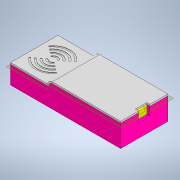
# Autodesk Inventor part: Part1
Saved by Autodesk Inventor 2021 (Build 250183000, 183)
## iProperties
Created: 2026-03-20
Part Number: Part1
Material: Generic
Document SubType Name: Modeling
Designer: Ignacio
Density: 1 g/cm^3
Appearance: Default
Author: Ignacio
Autodesk Inventor part; units mm, degrees
ref_plane "YZ Plane" through (0, 0, 0) normal (1, 0, 0) x (0, 1, 0)
ref_plane "XZ Plane" through (0, 0, 0) normal (0, 1, 0) x (-1, 0, 0)
ref_plane "XY Plane" through (0, 0, 0) normal (0, 0, 1) x (1, 0, 0)
sketch "Sketch1" plane through (0, 0, 0) normal (0, 1, 0) x (-1, 0, 0)
  line L0 (0, 0) -> (51, 0)
  line L1 (51, 0) -> (51, -51)
  line L2 (51, -51) -> (0, -51)
  line L3 (0, -51) -> (0, 0)
  dimension "d0" = 51
  constraints: 8 end point, 2 parallel, 2 perpendicular, 1 horizontal
  measures "d0" distance of L0.end L1.end
extrude "Extrusion1" add sketch "Sketch1" along normal blind 1.6
sketch "Sketch2" plane through (0, 0, 0) normal (0, -1, 0) x (1, 0, 0)
  line L0 (-49, -2) -> (-2, -2)
  line L1 (-2, -2) -> (-2, -49)
  line L2 (-2, -49) -> (-49, -49)
  line L3 (-49, -49) -> (-49, -2)
  line L4 (-49, -2) -> (-2, -49) construction
  line L5 (-2, -2) -> (-49, -49) construction
  line L6 (0, 0) -> (0, -51) construction
  line L7 (0, -25.5) -> (-25.5, -25.5) construction
  line L8 (-25.5, -25.5) -> (-25.5, -51) construction
  line L9 (0, -51) -> (-51, -51) construction
  dimension "d3" = 2
  dimension "d4" = 2
  constraints: 16 end point, 4 midpoint, 3 perpendicular, 2 parallel, 1 horizontal
  measures "d3" distance between parallel lines of L6 L1
  measures "d4" distance between parallel lines of L9 L2
extrude "Extrusion2" add sketch "Sketch2" along normal blind 4
sketch "Sketch3" plane through (0, 0, 0) normal (1, 0, 0) x (0, 1, 0)
  line L0 (1.6, -51) -> (1.6, 0) projected
  line L1 (1.6, -9.85) -> (16.1, -9.85)
  line L2 (16.1, -9.85) -> (16.1, -41.15)
  line L3 (16.1, -41.15) -> (1.6, -41.15)
  line L4 (1.6, -41.15) -> (1.6, -9.85)
  line L5 (1.6, -25.5) -> (16.1, -25.5) construction
  point P0 (0, 0)
  point P1 (1.6, -41.15)
  dimension "d7" = 14.5
  dimension "d8" = 31.3
  constraints: 10 end point, 3 midpoint, 2 parallel, 1 horizontal, 1 perpendicular, 1 point on line
  measures "d7" distance of L2.end L3.end
  measures "d8" distance of L1.end L2.end
extrude "Extrusion3" add sketch "Sketch3" along normal blind 15.4 and the other way blind 42
sketch "Sketch4" plane through (15.4, 0, 0) normal (1, 0, 0) x (0, 0, -1)
  line L0 (21.5, 14.1) -> (29.5, 14.1)
  line L1 (29.5, 14.1) -> (29.5, 18.1)
  line L2 (29.5, 18.1) -> (21.5, 18.1)
  line L3 (21.5, 18.1) -> (21.5, 14.1)
  line L4 (9.85, 16.1) -> (41.15, 16.1) projected
  line L5 (21.5, 14.1) -> (29.5, 18.1) construction
  line L6 (29.5, 14.1) -> (21.5, 18.1) construction
  point P0 (0, 0)
  point P1 (25.5, 16.1)
  dimension "d13" = 8
  dimension "d14" = 4
  constraints: 12 end point, 3 midpoint, 2 parallel, 1 horizontal, 1 perpendicular
  measures "d13" distance of L1.end L2.end
  measures "d14" distance of L0.end L1.end
extrude "Extrusion4" add sketch "Sketch4" along normal blind 1.5 and the other way blind 3
sketch "Sketch5" plane through (0, 1.6, 0) normal (0, 1, 0) x (1, 0, 0)
  line L0 (-49, 49) -> (-49, 2) projected
  line L1 (-48, 5.5) -> (-49, 5.5)
  line L2 (-49, 5.5) -> (-49, 45.5)
  line L3 (-49, 45.5) -> (-48, 45.5)
  line L4 (-48, 45.5) -> (-48, 5.5)
  line L5 (-51, 51) -> (-51, 0) projected
  line L6 (-51, 25.5) -> (-49, 25.5) construction
  point P0 (0, 0)
  dimension "d20" = 1
  dimension "d21" = 40
  constraints: 10 end point, 2 midpoint, 2 parallel, 2 perpendicular, 1 horizontal, 1 point on line
  measures "d20" distance of L1.start L1.end
  measures "d21" distance of L3.end L1.start
extrude "Extrusion5" add sketch "Sketch5" along normal blind 13
sketch "Sketch6" plane through (-49, 1.6, -45.5) normal (-1, 0, 0) x (0, 0, 1)
  line L0 (40, 0) -> (40, 13) projected
  line L1 (0, 13) -> (40, 13)
  line L2 (40, 13) -> (40, 11.5)
  line L3 (40, 11.5) -> (0, 11.5)
  line L4 (0, 11.5) -> (0, 13)
  point P0 (45.5, -1.6)
  dimension "d24" = 1.5
  constraints: 8 end point, 2 parallel, 1 horizontal, 1 perpendicular, 1 point on line
  measures "d24" distance between parallel lines of L1 L3
extrude "Extrusion6" add sketch "Sketch6" along normal blind 60
sketch "Sketch7" plane through (0, -4, 0) normal (0, -1, 0) x (1, 0, 0)
  line L0 (20.4, -54.3) -> (-114, -54.3)
  line L1 (-114, -54.3) -> (-114, 3.3)
  line L2 (-114, 3.3) -> (20.4, 3.3)
  line L3 (20.4, 3.3) -> (20.4, -54.3)
  line L4 (-49, -49) -> (-49, -2) projected
  line L5 (-49, -2) -> (-2, -2) projected
  line L6 (-2, -2) -> (-2, -49) projected
  line L7 (-2, -49) -> (-49, -49) projected
  line L8 (-51, 0) -> (0, 0) projected
  line L9 (0, -51) -> (-51, -51) projected
  line L10 (-109, -45.5) -> (-109, -5.5) projected
  line L11 (15.4, -9.85) -> (15.4, -41.15) projected
  dimension "d27" = 3.3
  dimension "d28" = 3.3
  dimension "d29" = 5
  dimension "d30" = 5
  constraints: 8 end point, 2 parallel, 1 horizontal, 1 perpendicular
  measures "d27" distance between parallel lines of L8 L2
  measures "d28" distance between parallel lines of L0 L9
  measures "d29" distance between parallel lines of L1 L10
  measures "d30" distance between parallel lines of L11 L3
extrude "Extrusion7" add sketch "Sketch7" along normal blind 3 separate body contours L0 L1 L2 L3 | L4 L5 L6 L7
sketch "Sketch8" plane through (0, -4, 0) normal (0, 1, 0) x (1, 0, 0)
  line L0 (20.4, -3.3) -> (-114, -3.3) projected
  line L1 (-114, -3.3) -> (-114, 54.3) projected
  line L2 (20.4, -3.3) -> (-114, -3.3)
  line L3 (-114, -3.3) -> (-114, 54.3)
  line L4 (-114, 54.3) -> (20.4, 54.3)
  line L5 (20.4, 54.3) -> (20.4, -3.3)
  line L6 (-110, 51.3) -> (16.4, 51.3)
  line L7 (16.4, 51.3) -> (16.4, -0.3)
  line L8 (16.4, -0.3) -> (-110, -0.3)
  line L9 (-110, -0.3) -> (-110, 51.3)
  line L10 (20.4, 54.3) -> (20.4, -3.3) projected
  line L11 (16.4, 20) -> (20.4, 20)
  line L12 (20.4, 20) -> (20.4, 31)
  line L13 (20.4, 31) -> (16.4, 31)
  line L14 (16.4, 31) -> (16.4, 20)
  line L15 (15.4, 21.5) -> (15.4, 9.85) projected
  line L16 (-109, 5.5) -> (-109, 45.5) projected
  line L17 (-51, 0) -> (0, 0) projected
  line L18 (0, 51) -> (-51, 51) projected
  line L19 (16.9, 21.5) -> (12.4, 21.5) projected
  line L20 (16.9, 21.5) -> (16.9, 29.5) projected
  line L21 (16.9, 25.5) -> (20.4, 25.5) construction
  dimension "d35" = 1
  dimension "d36" = 1
  dimension "d37" = 0.3
  dimension "d38" = 0.3
  dimension "d39" = 3
  dimension "d41" = 11
  constraints: 26 end point, 6 parallel, 4 perpendicular, 3 horizontal, 2 midpoint, 2 point on line
  measures "d35" distance between parallel lines of L15 L7
  measures "d36" distance between parallel lines of L9 L16
  measures "d37" distance between parallel lines of L17 L8
  measures "d38" distance between parallel lines of L18 L6
  measures "d39" distance between parallel lines of L8 L0
  measures "d41" distance between parallel lines of L13 L11
extrude "Extrusion8" add sketch "Sketch8" along normal blind 24 contours L0 L1 L4 L5 L13 L7 L6 L9 L8 L11 | L11 L7 L13 L5 bodies 2
sketch "Sketch9" plane through (20.4, -7, -54.3) normal (0, 0, -1) x (-1, 0, 0)
  line L0 (68.4, 21.6) -> (129.4, 21.6) construction
  line L1 (68.4, 21.6) -> (129.4, 21.6) construction
  line L2 (62.4, 21.85) -> (129.4, 21.85)
  arc A0 (87.4, 23.5667) -> (89.4, 21.85) centre (89.4, 23.8734) ccw
  arc A1 (87.4, 23.5667) -> (83.4, 27) centre (83.4, 22.9532) ccw
  line L3 (0, 27) -> (134.4, 27) projected
  line L4 (62.4, 8.6) -> (62.4, 23.1) projected
  line L5 (62.4, 23.1) -> (62.4, 8.6) projected
  line L6 (129.4, 21.85) -> (134.4, 21.85)
  line L7 (134.4, 27) -> (134.4, 0) projected
  line L8 (134.4, 27) -> (134.4, 21.85)
  line L9 (129.4, 20.1) -> (129.4, 21.6) projected
  point P0 (20.4, 7)
  dimension "d44" = 0.25
  dimension "d61" = 40
  dimension "d62" = 2
  dimension "d63" = 4
  constraints: 6 end point, 4 point on circle, 3 point on line, 3 tangent, 2 centre point, 1 collinear, 1 horizontal, 1 parallel
  measures "d44" distance between parallel lines of L0 L2
  measures "d61" distance from line of L9 A0.end
  measures "d62" horizontal distance of A0.end A0.start
  measures "d63" horizontal distance of A0.start A1.end
extrude "Extrusion9" cut sketch "Sketch9" against normal blind 65 bodies 2
sketch "Sketch10" plane through (0, -4, 0) normal (0, 1, 0) x (1, 0, 0)
  circle A0 centre (-89, 25.5) radius 10
  line L0 (-109, 5.5) -> (-109, 45.5) projected
  line L1 (-109, 25.5) -> (-89, 25.5) construction
  point P0 (0, 0)
  dimension "d48" = 20
  dimension "d49" = 20
  constraints: 2 end point, 1 centre point, 1 midpoint, 1 perpendicular
  measures "d48" distance from line of L0 L1.end
  measures "d49" diameter of A0
extrude "Extrusion10" add sketch "Sketch10" along normal blind 17 bodies 2
fillet "Fillet1" radius 4.25 1 edges at (-99, -4, -25.5)
sketch "Sketch11" plane through (0, -4, 0) normal (0, 1, 0) x (1, 0, 0)
  line L0 (-49, 49) -> (-49, 2) projected
  line L1 (-49, 2) -> (-2, 2) projected
  line L2 (-2, 2) -> (-2, 49) projected
  line L3 (-2, 49) -> (-49, 49) projected
  line L4 (0, 51) -> (-51, 51) projected
  line L5 (0, 0) -> (0, 51) projected
  line L6 (-51, 0) -> (0, 0) projected
  line L7 (-51, 51) -> (-51, 0) projected
  line L8 (2, 53) -> (-53, 53)
  line L9 (-53, 53) -> (-53, -2)
  line L10 (-53, -2) -> (2, -2)
  line L11 (2, -2) -> (2, 53)
  dimension "d53" = 2
  constraints: 8 end point, 3 other
  measures "d53" distance between parallel lines of L5 L11
extrude "Extrusion11" add sketch "Sketch11" along normal up to surface (4 mm away) contours L5 L6 L7 L4 | L11 L10 L9 L8 bodies 2
sketch "Sketch12" plane through (-53, 0, 0.3) normal (0, 1, 0) x (1, 0, 0)
  line L0 (55, 0) -> (0, 0) projected
  line L1 (0, 51.6) -> (55, 51.6) projected
  line L2 (55, 0) -> (53.4, 0)
  line L3 (53.4, 0) -> (53.4, 51.6)
  line L4 (53.4, 51.6) -> (55, 51.6)
  line L5 (55, 51.6) -> (55, 0)
  line L6 (53, 0.3) -> (53, 10.15) projected
  line L7 (0, 0) -> (1.6, 0)
  line L8 (1.6, 0) -> (1.6, 51.6)
  line L9 (1.6, 51.6) -> (0, 51.6)
  line L10 (0, 51.6) -> (0, 0)
  line L11 (2, 51.3) -> (2, 0.3) projected
  point P0 (53.4, 0)
  point P1 (1.6, 0)
  dimension "d56" = 0.4
  dimension "d57" = 0.4
  constraints: 16 end point, 4 parallel, 2 horizontal, 2 perpendicular, 2 point on line
  measures "d56" distance between parallel lines of L6 L3
  measures "d57" distance between parallel lines of L8 L11
extrude "Extrusion12" add sketch "Sketch12" along normal blind 1.5 contours L0 L3 L1 L5 | L0 L10 L1 L8 bodies 2
sketch "Sketch13" plane through (20.4, -7, 3.3) normal (1, 0, 0) x (0, 0, -1)
  line L0 (24.8, 25.1) -> (24.8, 21.1) projected
  line L1 (24.8, 21.1) -> (32.8, 21.1) projected
  line L2 (32.8, 21.1) -> (32.8, 25.1) projected
  line L3 (32.8, 25.1) -> (24.8, 25.1) projected
  line L4 (21.8, 27) -> (35.8, 27)
  line L5 (35.8, 27) -> (35.8, 16.1)
  line L6 (35.8, 16.1) -> (21.8, 16.1)
  line L7 (21.8, 16.1) -> (21.8, 27)
  line L8 (0, 27) -> (57.6, 27) projected
  line L9 (32.8, 25.1) -> (24.8, 25.1) construction
  line L10 (28.8, 25.1) -> (28.8, 27) construction
  point P0 (3.3, 7)
  point P1 (28.8, 16.1)
  dimension "d64" = 0
  dimension "d65" = 14
  dimension "d66" = 5
  constraints: 10 end point, 3 midpoint, 2 parallel, 1 horizontal, 1 perpendicular, 1 point on line
  measures "d64" distance between parallel lines of L8 L4
  measures "d65" distance of L5.end L6.end
  measures "d66" distance between parallel lines of L1 L6
extrude "Extrusion13" cut sketch "Sketch13" against normal blind 16.5 contours L3 L2 L1 L0 | L4 L5 L6 L7 bodies 2
thicken "Thicken1" operation new thickness 2 both sides no extend neighbours no toward (0, 1, 0) faces at (-8.7333, 20, 2.3) (-65.8693, 18.8069, 1.3) (-68.6824, 14.8751, 2.3) (-112.6667, 14.85, -34.1) (-68.8407, 14.8563, -52.3) (-66.6127, 17.7767, -53.3) (-8.7333, 20, -53.3)
move faces "Move1" translate (0, 0, -51.6) faces at (-10.0667, 21.3333, 0.3) (-65.8451, 20.478, 0.3) (-68.842, 15.5354, 0.3) (-96.3333, 15.5167, 0.3)
ref_plane "Work Plane1" through (-63, 18, 3.3) normal (0, -1, 0) x (1, 0, 0)
ref_plane "Work Plane2" through (-114, 12.85, 3.3) normal (0, -1, 0) x (1, 0, 0)
sketch "Sketch14" plane through (-114, 14.85, 3.3) normal (0, -1, 0) x (1, 0, 0)
  line L0 (45, -57.6) -> (45, 0) construction
  line L1 (45, 0) -> (0, 0) construction
  line L2 (0, 0) -> (0, -57.6) construction
  line L3 (0, -57.6) -> (45, -57.6) construction
  line L4 (4, -3) -> (45, -3) construction
  line L5 (4, -54.6) -> (4, -3) construction
  line L6 (45, -54.6) -> (4, -54.6) construction
  line L7 (45, -57.6) -> (45, -54.6) construction
  line L8 (0, -57.6) -> (45, -57.6) construction
  line L9 (0, 0) -> (0, -57.6) construction
  line L10 (45, 0) -> (0, 0) construction
  line L11 (45, -3) -> (45, 0) construction
  line L12 (45.25, -3.25) -> (4.25, -3.25) construction
  line L13 (4.25, -3.25) -> (4.25, -54.35) construction
  line L14 (4.25, -54.35) -> (45.25, -54.35) construction
  line L15 (45.25, -54.35) -> (45.25, -57.85) construction
  line L16 (45.25, -57.85) -> (-0.25, -57.85) construction
  line L17 (-0.25, -57.85) -> (-0.25, 0.25) construction
  line L18 (-0.25, 0.25) -> (45.25, 0.25) construction
  line L19 (45.25, 0.25) -> (45.25, -3.25) construction
  line L20 (45, -57.6) -> (45, 0) construction
  line L21 (4.25, -5.25) -> (45, -5.25)
  line L22 (45, -5.25) -> (45, -51.8103)
  line L23 (4.25, -3.25) -> (45, -3.25)
  line L24 (45, -3.25) -> (45, -5.25)
  line L25 (45, -5.25) -> (4.25, -5.25)
  line L26 (4.25, -5.25) -> (4.25, -3.25)
  line L27 (45, -54.35) -> (4.25, -54.35)
  line L28 (4.25, -54.35) -> (4.25, -52.35)
  line L29 (4.25, -52.35) -> (45, -52.35)
  line L30 (45, -52.35) -> (45, -54.35)
  point P0 (114, -3.3)
  point P1 (4.25, -5.25)
  dimension "d76" = 0.25
  dimension "d77" = 2
  dimension "d78" = 2
  constraints: 36 end point, 5 point on line, 4 parallel, 3 horizontal, 3 perpendicular, 7 other
  measures "d76" distance between parallel lines of L4 L12
  measures "d77" distance between parallel lines of L21 L12
  measures "d78" distance between parallel lines of L27 L29
extrude "Extrusion14" add sketch "Sketch14" along normal blind 3 bodies 3
chamfer "Chamfer1" distance 3 angle 45 2 edges at (-89.375, 14.85, -1.95) (-89.375, 14.85, -49.05)
chamfer "Chamfer2" distance 0.5 angle 45 10 edges at (-89.375, 11.85, 0.05) (-89.375, 11.85, -51.05) (-109.75, 11.85, -49.05) (-109.75, 11.85, -50.05) (-109.75, 11.85, -1.95) (-109.75, 11.85, -0.95) (-69, 11.85, -1.95) (-69, 11.85, -0.95) (-69, 11.85, -49.05) (-69, 11.85, -50.05)
sketch "Sketch15" plane through (-63, 20, 3.3) normal (0, -1, 0) x (1, 0, 0)
  line L0 (-46.75, -54.35) -> (-6, -54.35) projected
  line L1 (-6.5, -52.35) -> (-46.25, -52.35) projected
  line L2 (0, -52.35) -> (79.1, -52.35)
  line L3 (79.1, -52.35) -> (79.1, -54.35)
  line L4 (79.1, -54.35) -> (0, -54.35)
  line L5 (0, -54.35) -> (0, -52.35)
  line L6 (0, 0) -> (0, -57.6) projected
  line L7 (79.4, -21.8) -> (79.4, -35.8) projected
  line L8 (-51, 0) -> (-51, -57.6) projected
  line L9 (-51, -28.8) -> (108.3978, -28.8)
  line L10 (0, -5.25) -> (79.1, -5.25)
  line L11 (79.1, -5.25) -> (79.1, -3.25)
  line L12 (79.1, -3.25) -> (0, -3.25)
  line L13 (0, -3.25) -> (0, -5.25)
  point P0 (63, -3.3)
  point P1 (0, -3.25)
  point P2 (0, -5.25)
  dimension "d87" = 0.3
  constraints: 18 end point, 4 symmetric about line, 3 collinear, 2 horizontal, 2 parallel, 1 midpoint, 1 perpendicular
  measures "d87" distance between parallel lines of L3 L7
extrude "Extrusion15" add sketch "Sketch15" along normal blind 3 bodies 3
chamfer "Chamfer3" distance 3 angle 45 2 edges at (-23.45, 20, -1.95) (-23.45, 20, -49.05)
chamfer "Chamfer4" distance 0.5 angle 45 10 edges at (-63, 17.0001, -49.05) (-63, 17, -50.05) (-23.45, 17, -51.05) (16.1, 17.0001, -49.05) (16.1, 17, -50.05) (-63, 17.0001, -1.95) (-63, 17, -0.95) (-23.45, 17, 0.05) (16.1, 17.0001, -1.95) (16.1, 17, -0.95)
sketch "Sketch16" plane through (-114, 16.85, -54.3) normal (0, 1, 0) x (1, 0, 0)
  line L0 (45, 0) -> (45, -57.6) projected
  line L1 (0, 0) -> (45, 0) projected
  line L2 (0, -57.6) -> (0, 0) projected
  line L3 (45, -57.6) -> (0, -57.6) projected
  circle A0 centre (22.5116, -28.8) radius 20 construction
  circle A1 centre (22.5116, -28.8) radius 15 construction
  circle A2 centre (22.5116, -28.8) radius 10 construction
  circle A3 centre (22.5116, -28.8) radius 5 construction
  line L4 (38.3786, -40.9752) -> (6.6445, -16.6248) construction
  line L5 (38.3786, -16.6248) -> (6.6445, -40.9752) construction
  line L6 (45.0231, 0) -> (0, 0) construction
  line L7 (0, 0) -> (0, -57.6) construction
  line L8 (0, -57.6) -> (45.0231, -57.6) construction
  line L9 (45.0231, -57.6) -> (45.0231, 0) construction
  line L10 (45.0231, 0) -> (0, -57.6) construction
  line L11 (0, 0) -> (45.0231, -57.6) construction
  line L12 (22.5116, -28.8) -> (45, -28.8) construction
  line L13 (45, -8.25) -> (45, -49.35) construction
  arc A4 (6.6445, -40.9752) -> (38.3786, -40.9752) centre (22.5116, -28.8) ccw construction
  arc A5 (5.8511, -41.584) -> (39.172, -41.584) centre (22.5116, -28.8) ccw
  arc A6 (7.4378, -40.3665) -> (37.5853, -40.3665) centre (22.5116, -28.8) ccw
  arc A7 (7.4378, -40.3665) -> (5.8511, -41.584) centre (6.6445, -40.9752) ccw
  arc A8 (39.172, -41.584) -> (37.5853, -40.3665) centre (38.3786, -40.9752) ccw
  arc A9 (10.6113, -37.9314) -> (34.4119, -37.9314) centre (22.5116, -28.8) ccw construction
  arc A10 (9.8179, -38.5402) -> (35.2052, -38.5402) centre (22.5116, -28.8) ccw
  arc A11 (11.4046, -37.3227) -> (33.6185, -37.3227) centre (22.5116, -28.8) ccw
  arc A12 (11.4046, -37.3227) -> (9.8179, -38.5402) centre (10.6113, -37.9314) ccw
  arc A13 (35.2052, -38.5402) -> (33.6185, -37.3227) centre (34.4119, -37.9314) ccw
  arc A14 (14.578, -34.8876) -> (30.4451, -34.8876) centre (22.5116, -28.8) ccw construction
  arc A15 (13.7847, -35.4964) -> (31.2384, -35.4964) centre (22.5116, -28.8) ccw
  arc A16 (15.3714, -34.2789) -> (29.6517, -34.2789) centre (22.5116, -28.8) ccw
  arc A17 (15.3714, -34.2789) -> (13.7847, -35.4964) centre (14.578, -34.8876) ccw
  arc A18 (31.2384, -35.4964) -> (29.6517, -34.2789) centre (30.4451, -34.8876) ccw
  arc A19 (18.5448, -31.8438) -> (26.4783, -31.8438) centre (22.5116, -28.8) ccw construction
  arc A20 (17.7514, -32.4526) -> (27.2717, -32.4526) centre (22.5116, -28.8) ccw
  arc A21 (19.3381, -31.235) -> (25.685, -31.235) centre (22.5116, -28.8) ccw
  arc A22 (19.3381, -31.235) -> (17.7514, -32.4526) centre (18.5448, -31.8438) ccw
  arc A23 (27.2717, -32.4526) -> (25.685, -31.235) centre (26.4783, -31.8438) ccw
  arc A24 (26.4783, -25.7562) -> (18.5448, -25.7562) centre (22.5116, -28.8) ccw construction
  arc A25 (27.2717, -25.1474) -> (17.7514, -25.1474) centre (22.5116, -28.8) ccw
  arc A26 (25.685, -26.365) -> (19.3381, -26.365) centre (22.5116, -28.8) ccw
  arc A27 (25.685, -26.365) -> (27.2717, -25.1474) centre (26.4783, -25.7562) ccw
  arc A28 (17.7514, -25.1474) -> (19.3381, -26.365) centre (18.5448, -25.7562) ccw
  arc A29 (28.67, -20.9213) -> (14.578, -22.7124) centre (22.5116, -28.8) ccw construction
  arc A30 (31.2384, -22.1036) -> (13.7847, -22.1036) centre (22.5116, -28.8) ccw
  arc A31 (29.6517, -23.3211) -> (15.3714, -23.3211) centre (22.5116, -28.8) ccw
  arc A32 (29.6517, -23.3211) -> (31.2384, -22.1036) centre (30.4451, -22.7124) ccw
  arc A33 (13.7847, -22.1036) -> (15.3714, -23.3211) centre (14.578, -22.7124) ccw
  arc A34 (34.4119, -19.6686) -> (10.6113, -19.6686) centre (22.5116, -28.8) ccw construction
  arc A35 (35.2052, -19.0598) -> (9.8179, -19.0598) centre (22.5116, -28.8) ccw
  arc A36 (33.6185, -20.2773) -> (11.4046, -20.2773) centre (22.5116, -28.8) ccw
  arc A37 (33.6185, -20.2773) -> (35.2052, -19.0598) centre (34.4119, -19.6686) ccw
  arc A38 (9.8179, -19.0598) -> (11.4046, -20.2773) centre (10.6113, -19.6686) ccw
  arc A39 (38.3786, -16.6248) -> (6.6445, -16.6248) centre (22.5116, -28.8) ccw construction
  arc A40 (39.172, -16.016) -> (5.8511, -16.016) centre (22.5116, -28.8) ccw
  arc A41 (37.5853, -17.2335) -> (7.4378, -17.2335) centre (22.5116, -28.8) ccw
  arc A42 (37.5853, -17.2335) -> (39.172, -16.016) centre (38.3786, -16.6248) ccw
  arc A43 (5.8511, -16.016) -> (7.4378, -17.2335) centre (6.6445, -16.6248) ccw
  point P0 (114, -54.3)
  point P1 (22.5116, -28.8)
  dimension "d100" = 75
  dimension "d96" = 40
  dimension "d97" = 5
  dimension "d98" = 5
  dimension "d99" = 5
  dimension "d101" = 37.5
  dimension "d102" = 2
  dimension "d103" = 2
  dimension "d104" = 2
  dimension "d105" = 2
  dimension "d106" = 2
  dimension "d107" = 2
  dimension "d108" = 2
  dimension "d109" = 2
  constraints: 90 point on circle, 44 centre point, 32 tangent, 14 end point, 12 coincident, 4 midpoint, 2 parallel, 1 horizontal, 1 perpendicular, 21 other
  measures "d96" diameter of A0
  measures "d97" radial gap between concentric circles of A0 A1
  measures "d98" radial gap between concentric circles of A1 A2
  measures "d99" radial gap between concentric circles of A2 A3
  measures "d102" diameter of A7
  measures "d103" diameter of A12
  measures "d104" diameter of A17
  measures "d105" diameter of A22
  measures "d106" diameter of A28
  measures "d107" diameter of A33
  measures "d108" diameter of A38
  measures "d109" diameter of A43
extrude "Extrusion16" cut sketch "Sketch16" against normal blind 0.5 contours A7 A6 A8 A5 | A12 A11 A13 A10 | A17 A16 A18 A15 | A22 A21 A23 A20 | A27 A26 A28 A25 | A32 A31 A33 A30 | A37 A36 A38 A35 | A42 A41 A43 A40 bodies 3
equation "\"d28\" = d27"
equation "\"d57\" = d56"
equation "\"d97\" = d98"
equation "\"d98\" = d99"
equation "\"d101\" = 0.5 * d100"
body "Solid1"
body "Solid2"
body "Solid4"
